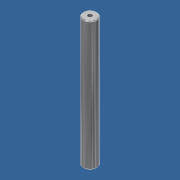
# Autodesk Inventor part: P1704_001
Saved by Autodesk Inventor 2015 SP2 (Build 190223200, 223)
## iProperties
Created: 2017-02-08
Part Number: P1704_001
Project: Manette arcade
Material: .EN AW-6082/AlMgSi1
Description: Pied
Document SubType Name: Modeling
Designer: Alexandre.PICOTTE
Authority: Ø8x75
Density: 2.7 g/cm^3
Appearance: Métal
Mass: 9.93821 g
Surface Area: 21.0302 cm^2
Volume: 3.68082 cm^3
Material number: ---
Author: Boris.GAUDARD
Autodesk Inventor part; units mm, degrees
ref_plane "Plan YZ" through (0, 0, 0) normal (1, 0, 0) x (0, 1, 0)
ref_plane "Plan XZ" through (0, 0, 0) normal (0, 1, 0) x (-1, 0, 0)
ref_plane "Plan XY" through (0, 0, 0) normal (0, 0, 1) x (1, 0, 0)
sketch "Esquisse1" plane through (0, 0, 0) normal (0, 0, 1) x (1, 0, 0)
  circle A0 centre (0, 0) radius 4
  dimension "d0" = 8
  constraints: 1 centre point, 1 coincident
  measures "d0" diameter of A0
extrude "Extrusion1" add sketch "Esquisse1" along normal blind 75
sketch "Esquisse6" plane through (0, 0, 75) normal (0, 0, 1) x (1, 0, 0)
  point P0 (0, 0)
  point P1 (0, 0)
  constraints: 1 coincident
hole "Perçage1" at (0, 0, 75) direction (0, 0, -1) diameter 2.459 depth 8.5 tip angle 118 thread size "M3x0.5" class "6H" standard "ISO M"
sketch "Esquisse7" plane through (0, 0, 0) normal (0, 0, -1) x (-1, 0, 0)
  circle A0 centre (0, 0) radius 1.2295 projected
  constraints: 1 coincident
hole "Perçage2" at (0, 0, 0) direction (0, 0, 1) diameter 2.459 depth 8.5 tip angle 118 thread size "M3x0.5" class "6H" standard "ISO M"
chamfer "Chanfrein1" distance 0.5 angle 45 2 edges at (-4, 0, 0) (-4, 0, 75)
